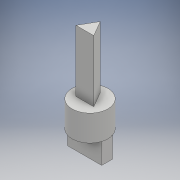
# Autodesk Inventor part: rotor
Saved by Autodesk Inventor 2017 (Build 210142000, 142)
## iProperties
Created: 2016-11-08
Part Number: rotor
Material: Generic
Document SubType Name: Modeling
Designer: Camilo
Density: 1 g/cm^3
Appearance: Default
Author: Camilo
Autodesk Inventor part; units mm, degrees
ref_plane "YZ Plane" through (0, 0, 0) normal (1, 0, 0) x (0, 1, 0)
ref_plane "XZ Plane" through (0, 0, 0) normal (0, 1, 0) x (-1, 0, 0)
sketch "Sketch1" plane through (0, 0, 0) normal (0, 0, 1) x (1, 0, 0)
  line L0 (-12.037, -14.2497) -> (-13.9713, -17.6) construction
  line L1 (-13.9713, -17.6) -> (-17.8398, -17.6) construction
  line L2 (-17.8398, -17.6) -> (-19.774, -14.2497) construction
  line L3 (-19.774, -14.2497) -> (-17.8398, -10.8995) construction
  line L4 (-17.8398, -10.8995) -> (-13.9713, -10.8995) construction
  line L5 (-13.9713, -10.8995) -> (-12.037, -14.2497) construction
  circle A0 centre (-15.9055, -14.2497) radius 28.486 construction
  line L6 (-12.1525, -14.2497) -> (-14.029, -17.5)
  line L7 (-14.029, -17.5) -> (-17.782, -17.5)
  line L8 (-17.782, -17.5) -> (-19.6585, -14.2497)
  line L9 (-19.6585, -14.2497) -> (-17.782, -10.9995)
  line L10 (-17.782, -10.9995) -> (-14.029, -10.9995) construction
  line L11 (-14.029, -10.9995) -> (-12.1525, -14.2497)
  line L12 (-15.9055, -10.7856) -> (-18.9055, -15.9818) construction
  line L13 (-18.9055, -15.9818) -> (-12.9055, -15.9818) construction
  line L14 (-12.9055, -15.9818) -> (-15.9055, -10.7856) construction
  line L15 (-15.9055, -11.0856) -> (-18.6457, -15.8318)
  line L16 (-18.6457, -15.8318) -> (-13.1653, -15.8318)
  line L17 (-13.1653, -15.8318) -> (-15.9055, -11.0856)
  point P0 (0, 0)
  dimension "d0" = 0.1
  dimension "d14" = 0.15
  constraints: 18 end point, 7 other
  measures "d0" distance between parallel lines of L4 L10
  measures "d14" distance between parallel lines of L14 L17
extrude "Extrusion1" add sketch "Sketch1" along normal blind 25
sketch "Sketch2" plane through (0, 0, 0) normal (0, 0, 1) x (1, 0, 0)
  circle A0 centre (-15.9055, -14.2497) radius 6 construction
  circle A1 centre (-15.9055, -14.2497) radius 5.5
  point P0 (0, 0)
  dimension "d3" = 0.5
  constraints: 1 centre point, 1 coincident
  measures "d3" radial gap between concentric circles of A0 A1
extrude "Extrusion2" add sketch "Sketch2" along normal blind 6
sketch "Sketch3" plane through (-15.9055, -14.2497, 0) normal (0, 0, -1) x (-1, 0, 0)
  circle A0 centre (0, 0) radius 5.5 projected
  point P0 (-15.9055, 14.2497)
ref_plane "Work Plane1" through (-52.6055, -32.2497, -2) normal (0, 0, 1) x (1, 0, 0)
extrude "Extrusion3" add sketch "Sketch3" along normal up to surface (2 mm away)
sketch "Sketch4" plane through (-15.9055, -14.2497, -2) normal (0, 0, -1) x (-1, 0, 0)
  circle A0 centre (0, 0) radius 5.5 projected
  circle A1 centre (0, 0) radius 5.5 projected
  line L0 (-5.2467, -1.65) -> (5.2467, -1.65)
  line L1 (5.2467, -1.65) -> (5.2467, 1.65)
  line L2 (5.2467, 1.65) -> (-5.2467, 1.65)
  line L3 (-5.2467, 1.65) -> (-5.2467, -1.65)
  line L4 (-5.2467, -1.65) -> (5.2467, 1.65) construction
  line L5 (5.2467, -1.65) -> (-5.2467, 1.65) construction
  point P0 (-15.9055, 14.2497)
  dimension "d8" = 3.3
  constraints: 12 end point, 2 midpoint, 2 parallel, 1 horizontal, 1 perpendicular, 2 other
  measures "d8" distance of L1.end L0.end
extrude "Extrusion4" add sketch "Sketch4" along normal blind 6.4 contours L1 L0 L3 L2
body "Solid1"
